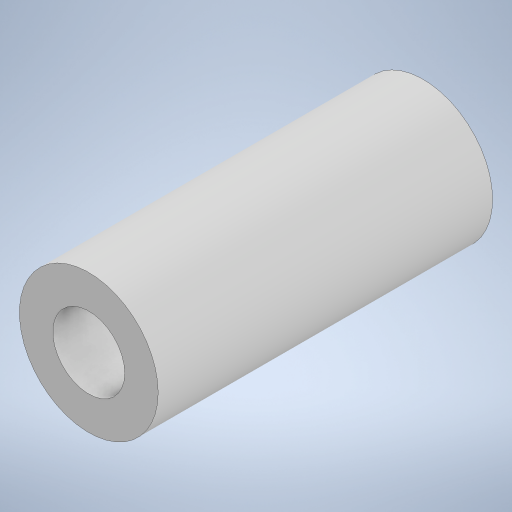
# Autodesk Inventor part: スペーサ20mm_内径3.3mm
Saved by Autodesk Inventor 2024.3 (Build 283343000, 343)
## iProperties
Created: 2024-10-09
Part Number: スペーサ20mm_内径3.3mm
Material: 一般
Document SubType Name: Modeling
Designer: hikou
Density: 1 g/cm^3
Appearance: 既定
Author: hikou
Autodesk Inventor part; units mm, degrees
ref_plane "YZ Plane" through (0, 0, 0) normal (1, 0, 0) x (0, 1, 0)
ref_plane "XZ Plane" through (0, 0, 0) normal (0, 1, 0) x (-1, 0, 0)
ref_plane "XY Plane" through (0, 0, 0) normal (0, 0, 1) x (1, 0, 0)
sketch "スケッチ1" plane through (0, 0, 0) normal (0, 0, 1) x (1, 0, 0)
  circle A0 centre (0, 0) radius 2.15
  circle A1 centre (0, 0) radius 4.15
  dimension "d0" = 4.3
  dimension "d1" = 8.3
  constraints: 2 centre point, 2 coincident
  measures "d0" diameter of A0
  measures "d1" diameter of A1
extrude "押し出し1" add sketch "スケッチ1" along normal mid plane 20
